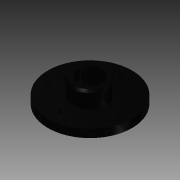
# Autodesk Inventor part: ServoHorn
Saved by Autodesk Inventor 2015 (Build 190159000, 159)
## iProperties
Created: 2015-10-11
Part Number: ServoHorn
Material: Generic
Document SubType Name: Modeling
Designer: styku
Density: 1 g/cm^3
Appearance: Fine Textured - Black
Mass: 0.769428 g
Surface Area: 10.7681 cm^2
Volume: 0.769428 cm^3
Author: styku
Autodesk Inventor part; units mm, degrees
ref_plane "YZ Plane" through (0, 0, 0) normal (1, 0, 0) x (0, 1, 0)
ref_plane "XZ Plane" through (0, 0, 0) normal (0, 1, 0) x (-1, 0, 0)
ref_plane "XY Plane" through (0, 0, 0) normal (0, 0, 1) x (1, 0, 0)
sketch "Sketch1" plane through (0, 0, 0) normal (0, 0, 1) x (1, 0, 0)
  circle A0 centre (0, 0) radius 10.5
  circle A1 centre (0, 0) radius 4.5
  circle A2 centre (0, 0) radius 3
  line L0 (-15, 0) -> (15, 0) construction
  line L1 (0, -19) -> (0, 21.6238) construction
  circle A3 centre (0, -7.5) radius 0.5
  circle A4 centre (0, 7.5) radius 0.5
  circle A5 centre (0, 0) radius 1
  circle A6 centre (0, 0) radius 2.5
  dimension "d0" = 21
  dimension "d1" = 9
  dimension "d2" = 6
  dimension "d3" = 1
  dimension "d4" = 7.5
  dimension "d5" = 2
  dimension "d6" = 5
  constraints: 7 centre point, 5 coincident, 4 end point, 2 midpoint, 2 point on line, 2 vertical, 1 horizontal, 1 symmetric about line, 1 other
  measures "d0" diameter of A0
  measures "d1" diameter of A1
  measures "d2" diameter of A2
  measures "d3" diameter of A3
  measures "d4" distance of point (0, 0) A3.centre
  measures "d5" diameter of A5
  measures "d6" diameter of A6
extrude "Extrusion1" add sketch "Sketch1" along normal blind 6 contours A1
extrude "Extrusion2" add sketch "Sketch1" along normal blind 2 contours A0 | A2 | A6
extrude "Extrusion3" cut sketch "Sketch1" along normal blind 1 contours A1 | A6
chamfer "Chamfer1" distance 0.5 angle 45 1 edges at (-4.5, 0, 6)
body "Solid1"
